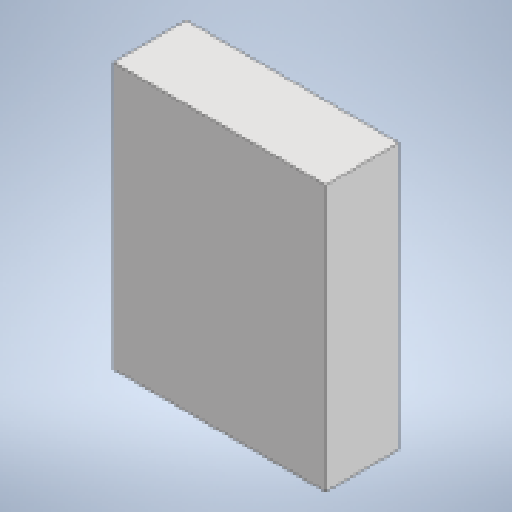
# Autodesk Inventor part: BSH 01 bag
Saved by Autodesk Inventor 2025 (Build 290162010, 162A)
## iProperties
Created: 2024-08-27
Part Number: BSH 01 bag
Material: Generic
Document SubType Name: Modeling
Designer: DELL
Density: 1 g/cm^3
Appearance: Default
Author: DELL
Autodesk Inventor part; units mm, degrees
ref_plane "YZ Plane" through (0, 0, 0) normal (1, 0, 0) x (0, 1, 0)
ref_plane "XZ Plane" through (0, 0, 0) normal (0, 1, 0) x (-1, 0, 0)
ref_plane "XY Plane" through (0, 0, 0) normal (0, 0, 1) x (1, 0, 0)
sketch "Sketch1" plane through (0, 0, 0) normal (0, 0, 1) x (1, 0, 0)
  line L0 (800, 275) -> (-800, 275)
  line L1 (-800, 275) -> (-800, -275)
  line L2 (-800, -275) -> (800, -275)
  line L3 (800, -275) -> (800, 275)
  line L4 (800, 275) -> (-800, -275) construction
  line L5 (-800, 275) -> (800, -275) construction
  point P0 (0, 0)
  dimension "d0" = 1600
  dimension "d1" = 550
  constraints: 12 end point, 2 midpoint, 2 parallel, 1 horizontal, 1 perpendicular
  measures "d0" distance of L2.end L1.end
  measures "d1" distance of L1.end L0.end
extrude "Extrusion1" add sketch "Sketch1" along normal blind 2000
body "Solid1"
